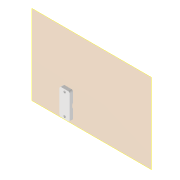
# Autodesk Inventor part: 20_M12_Lens_Fixation_1
Saved by Autodesk Inventor 2022 (Build 260153000, 153)
## iProperties
Created: 2022-09-19
Part Number: 20_M12_Lens_Fixation_1
Material: Generisch
Document SubType Name: Modeling
Designer: UC2
Density: 1 g/cm^3
Appearance: Vorgabe
Author: UC2
Autodesk Inventor part; units mm, degrees
ref_plane "YZ Plane" through (0, 0, 0) normal (1, 0, 0) x (0, 1, 0)
ref_plane "XZ Plane" through (0, 0, 0) normal (0, 1, 0) x (-1, 0, 0)
ref_plane "XY Plane" through (0, 0, 0) normal (0, 0, 1) x (1, 0, 0)
ref_plane "Arbeitsebene1" through (0, 0, 0) normal (0, 0, 1) x (1, 0, 0)
sketch "Skizze1" plane through (0, 0, 0) normal (0, 0, 1) x (1, 0, 0)
  circle A0 centre (-27.8589, -14.9953) radius 1.4 projected
  circle A1 centre (-27.8589, -39.949) radius 1.4 projected
  line L0 (-21.8589, -42.949) -> (-33.8589, -42.949)
  line L1 (-33.8589, -42.949) -> (-33.8589, -11.9953)
  line L2 (-33.8589, -11.9953) -> (-21.8589, -11.9953)
  line L3 (-21.8589, -11.9953) -> (-21.8589, -42.949)
  line L4 (-21.8589, -42.949) -> (-33.8589, -11.9953) construction
  line L5 (-33.8589, -42.949) -> (-21.8589, -11.9953) construction
  line L6 (-59.9, -42.75) -> (59.9, -42.75) projected
  point P0 (0, 0)
  point P1 (-27.8589, -27.4722)
  point P2 (-33.8589, -42.75)
  point P3 (-21.8589, -42.75)
  dimension "d0" = 24.9538
  dimension "d1" = 3
  dimension "d2" = 3
  dimension "d3" = 12
  constraints: 12 end point, 2 midpoint, 2 parallel, 1 horizontal, 1 perpendicular
  measures "d0" distance of A1.centre A0.centre
  measures "d1" distance from line of A0.centre L2
  measures "d2" distance from line of L0 A1.centre
  measures "d3" distance between parallel lines of L3 L1
extrude "Extrusion1" add sketch "Skizze1" along normal blind 4 contours L6 L1 L2 L3
fillet "Rundung1" radius 2 4 edges at (-21.8589, -11.9953, 2) (-33.8589, -11.9953, 2) (-21.8589, -42.75, 2) (-33.8589, -42.75, 2)
sketch "Skizze2" plane through (-21.8589, -40.75, 0) normal (1, 0, 0) x (0, 0, -1)
  circle A0 centre (4.8526, 13) radius 4.7625 projected
  circle A1 centre (4.3786, 13) radius 5.5
  point P0 (0, 40.75)
  dimension "d7" = 11
  constraints: 1 centre point
  measures "d7" diameter of A1
extrude "Extrusion2" cut sketch "Skizze2" against normal through all contours A0 | A1
